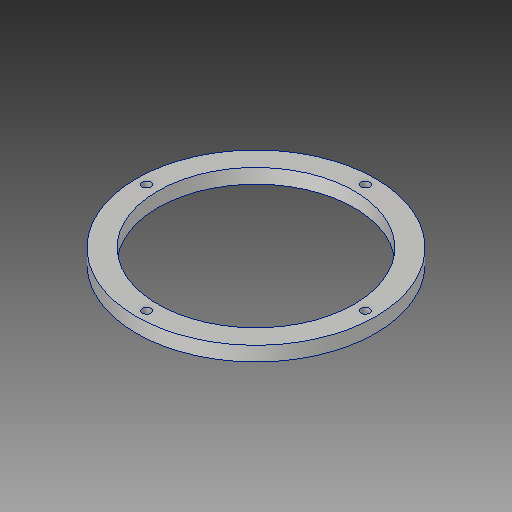
# Autodesk Inventor part: turntable2
Saved by Autodesk Inventor 2019 (Build 230136000, 136)
## iProperties
Created: 2018-11-14
Part Number: turntable2
Material: アルミニウム 6061
Document SubType Name: Modeling
Designer: miyas
Density: 2.7 g/cm^3
Appearance: アルミニウム - フラット
Mass: 113.106 g
Surface Area: 172.002 cm^2
Volume: 41.8912 cm^3
Author: miyas
Autodesk Inventor part; units mm, degrees
ref_plane "YZ Plane" through (0, 0, 0) normal (1, 0, 0) x (0, 1, 0)
ref_plane "XZ Plane" through (0, 0, 0) normal (0, 1, 0) x (-1, 0, 0)
ref_plane "XY Plane" through (0, 0, 0) normal (0, 0, 1) x (1, 0, 0)
sketch "スケッチ1" plane through (0, 0, 0) normal (0, 1, 0) x (-1, 0, 0)
  circle A0 centre (0, 0) radius 57.5
  circle A1 centre (0, 0) radius 70
  dimension "d0" = 115
  dimension "d1" = 140
  constraints: 2 centre point, 2 coincident
  measures "d0" diameter of A0
  measures "d1" diameter of A1
extrude "押し出し1" add sketch "スケッチ1" along normal blind 8.5
sketch "スケッチ2" plane through (0, 8.5, 0) normal (0, 1, 0) x (1, 0, 0)
  point P0 (0, 0)
  point P1 (0, 64)
  point P2 (-64, 0)
  point P3 (0, -64)
  point P4 (64, 0)
  dimension "d4" = 64
  dimension "d7" = 360
  constraints: 1 vertical alignment, 5 other
  measures "d4" distance of point (0, 0) point (0, 64)
hole "穴1" at (0, 8.5, -64) at (-64, 8.5, 0) at (0, 8.5, 64) at (64, 8.5, 0) direction (0, -1, 0) diameter 5 end through all
